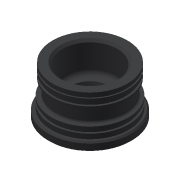
# Autodesk Inventor part: Cavity-middle
Saved by Autodesk Inventor 2022 Beta2 (Build 260130000, 130) ContinuousBuild 0
## iProperties
Shininess: 64.0
Length Units: 11269
Angle Units: 11279
Time Units: 11290
Mass Units: 11283
Length Display Precision: 3
Angle Display Precision: 2
Compacted: True
Part Number: Cavity-middle
Document SubType Name: Modeling
Created: 2003-04-07
Designer: demo
Density: 1 g/cm^3
Material: Generic
Appearance: Generic
Density: 0.0
Volumn: 0.0
Area: 0.0
PropertySet Name: Model Information
Control State: 0
Master: False
Checked Out: False
Author: demo
Autodesk Inventor part; units mm, degrees
ref_plane "YZ Plane" through (0, 0, 0) normal (1, 0, 0) x (0, 1, 0)
sketch "Sketch1" plane through (0, 0, 0) normal (0, 0, 1) x (1, 0, 0)
  line L0 (2.381, 29.408) -> (2.381, -22.2008)
  line L1 (-18.8276, 20.7851) -> (-24.5938, 20.7851)
  line L2 (-24.5938, 20.7851) -> (-24.5938, 18.3721)
  line L3 (-24.5938, 18.3721) -> (-23.654, 18.3721)
  line L4 (-23.654, 18.3721) -> (-23.654, 16.9751)
  line L5 (-23.654, 16.9751) -> (-24.5938, 16.9751)
  line L6 (-24.5938, 16.9751) -> (-24.5938, 14.4351)
  line L7 (-24.5938, 14.4351) -> (-23.1968, 14.4351)
  line L8 (-23.1968, 14.4351) -> (-23.1968, 12.1491)
  line L9 (-23.1968, 12.1491) -> (-24.5938, 12.1491)
  line L10 (-24.5938, 12.1491) -> (-24.5938, 10.6251)
  line L11 (-24.5938, 10.6251) -> (-23.8268, 10.6251)
  line L12 (-22.2393, 9.0376) -> (-22.2393, 1.6716)
  line L13 (-23.8268, 0.0841) -> (-25.3635, 0.0841)
  line L14 (-25.3635, 0.0841) -> (-25.3635, -2.0749)
  line L15 (-25.3635, -2.0749) -> (-23.9919, -2.0749)
  line L16 (-23.9919, -2.0749) -> (-23.9919, -4.3609)
  line L17 (-23.9919, -4.3609) -> (-25.3635, -4.3609)
  line L18 (-25.3635, -4.3609) -> (-25.3635, -7.8153)
  line L19 (-25.3635, -7.8153) -> (-26.7351, -7.8153)
  line L20 (-27.7511, -8.8313) -> (-27.7511, -13.1493)
  line L21 (-26.7351, -14.1653) -> (-7.6089, -14.1653)
  line L22 (-7.6089, -14.1653) -> (-11.1851, -0.8186)
  line L23 (-11.1851, -0.8186) -> (-14.1061, -0.8186)
  line L24 (-17.2811, 2.3564) -> (-17.2811, 19.1712)
  line L25 (-17.2811, 19.1712) -> (-18.8276, 20.7851)
  arc A0 (-17.2811, 2.3564) -> (-14.1061, -0.8186) centre (-14.1061, 2.3564) ccw
  arc A1 (-22.2393, 9.0376) -> (-23.8268, 10.6251) centre (-23.8268, 9.0376) ccw
  arc A2 (-23.8268, 0.0841) -> (-22.2393, 1.6716) centre (-23.8268, 1.6716) ccw
  line L26 (-27.7511, -8.8313) -> (-26.7351, -7.8153)
  line L27 (-27.7511, -13.1493) -> (-26.7351, -14.1653)
  point P0 (-27.7511, -7.8153)
  point P1 (-27.7511, -14.1653)
  dimension "d0" = 3.175
  dimension "d1" = 1.5875
  dimension "d2" = 1.016
  dimension "d3" = 1.016
  dimension "d4" = 1.016
  dimension "d5" = 1.016
  constraints: 56 end point, 14 parallel, 6 perpendicular, 6 point on circle, 6 tangent, 5 point on line, 3 centre point, 2 collinear, 1 equal radius, 1 vertical
  measures "d0" radius of A0
  measures "d1" radius of A1
  measures "d2" distance of L20.start point (-27.751, -7.815)
  measures "d3" distance of L19.end point (-27.751, -7.815)
  measures "d4" distance of L20.end point (-27.751, -14.165)
  measures "d5" distance of L21.start point (-27.751, -14.165)
revolve "Revolution1" add sketch "Sketch1" angle 360 about axis through (2.381, 29.408, 0) along (0, -1, 0)
ref_plane "Work Plane1" through (2.381, -7.4919, 0) normal (0, 0, -1) x (0, 1, 0)
ref_plane "Work Plane2" through (2.381, -7.4919, 0) normal (1, 0, 0) x (0, 1, 0)
sketch "Sketch2" plane through (2.381, -14.1653, 0) normal (0, -1, 0) x (1, 0, 0)
  circle A0 centre (0, 0) radius 9.9898 projected
  circle A1 centre (0, 0) radius 13.97
  line L0 (48.2112, 0) -> (-36.1584, 0) projected
  dimension "d7" = 27.94
  constraints: 1 centre point, 1 coincident, 1 concentric
  measures "d7" diameter of A1
sketch "Sketch3" plane through (2.381, -7.4919, 0) normal (0, 0, -1) x (0, 1, 0)
  line L0 (-10.1684, 0) -> (38.7621, 0) projected
  line L1 (-6.6734, -29.116) -> (-6.6734, 29.116) projected
  circle A0 centre (-7.7529, -13.97) radius 2.273
  line L2 (-10.1684, 0) -> (38.7621, 0) projected
  dimension "d9" = 1.0795
  dimension "d10" = 13.97
  constraints: 1 centre point
  measures "d9" distance from line of L1 A0.centre
  measures "d10" distance from line of L0 A0.centre
sweep "Sweep1" cut profiles "Sketch3" path "Sketch2" path curves A1
equation "\"d4\" = d2"
equation "\"d5\" = d3"
body "Solid1"
